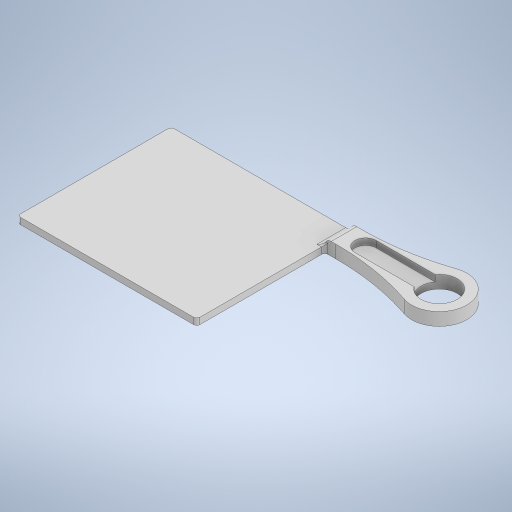
# Autodesk Inventor part: wachlarz
Saved by Autodesk Inventor 2023 (Build 270158000, 158)
## iProperties
Created: 2024-05-14
Part Number: wachlarz
Material: Ogólny
Document SubType Name: Modeling
Designer: kamil
Density: 1 g/cm^3
Appearance: Domyślna
Author: kamil
Autodesk Inventor part; units mm, degrees
ref_plane "YZ Plane" through (0, 0, 0) normal (1, 0, 0) x (0, 1, 0)
ref_plane "XZ Plane" through (0, 0, 0) normal (0, 1, 0) x (-1, 0, 0)
ref_plane "XY Plane" through (0, 0, 0) normal (0, 0, 1) x (1, 0, 0)
sketch "Szkic1" plane through (0, 0, 0) normal (0, 1, 0) x (-1, 0, 0)
  circle A0 centre (0, 0) radius 2.815
  circle A1 centre (0, 0) radius 4.315
  line L0 (43.875, 2) -> (0, 2)
  line L1 (0, 2) -> (0, -2)
  line L2 (0, -2) -> (43.875, -2)
  line L3 (43.875, -2) -> (43.875, 2)
  point P0 (43.875, 0)
  point P1 (3.8235, 2)
  point P2 (3.8235, -2)
  dimension "d0" = 5.63
  dimension "d2" = 1.5
  dimension "d5" = 43.875
  dimension "d6" = 4
  constraints: 8 end point, 2 centre point, 2 parallel, 1 coincident, 1 horizontal, 1 horizontal alignment, 1 midpoint, 1 perpendicular, 1 vertical alignment
  measures "d0" diameter of A0
  measures "d2" radial gap between concentric circles of A0 A1
  measures "d5" distance of L2.end L1.end
  measures "d6" distance of L1.end L0.end
extrude "Wyciągnięcie proste1" add sketch "Szkic1" along normal blind 2 contours A0 L0 A1 L2 | A0 L2 A1 L0 | L0 L3 L2 A1
sketch "Szkic2" plane through (0, 2, 0) normal (0, 1, 0) x (1, 0, 0)
  line L0 (-43.875, -2) -> (-3.8235, -2) projected
  arc A0 (-3.8235, -2) -> (-3.8235, 2) centre (0, 0) ccw projected
  line L1 (-3.8235, 2) -> (-43.875, 2) projected
  line L2 (-43.875, 2) -> (-43.875, -2) projected
  circle A1 centre (0, 0) radius 2.815 projected
  line L3 (-43.875, -2) -> (-15.875, -2)
  line L4 (-15.875, -2) -> (-15.875, -22)
  line L5 (-15.875, -22) -> (-43.875, -22)
  line L6 (-43.875, -22) -> (-43.875, -2)
  point P0 (-15.875, -2)
  dimension "d9" = 28
  dimension "d10" = 20
  constraints: 8 end point, 2 parallel, 1 horizontal, 1 perpendicular
  measures "d9" distance of L4.end L5.end
  measures "d10" distance of L3.end L4.end
extrude "Wyciągnięcie proste2" add sketch "Szkic2" against normal blind 2 contours L0 L4 L5 L6
sketch "Szkic3" plane through (0, 2, 0) normal (0, 1, 0) x (1, 0, 0)
  line L0 (0, 0) -> (-11.5, 0) construction
  line L1 (0, 1.65) -> (-11.5, 1.65)
  line L2 (-11.5, -1.65) -> (0, -1.65)
  arc A0 (0, -1.65) -> (0, 1.65) centre (0, 0) ccw
  arc A1 (-11.5, 1.65) -> (-11.5, -1.65) centre (-11.5, 0) ccw
  point P0 (-5.75, 0)
  dimension "d13" = 11.5
  dimension "d14" = 3.3
  constraints: 8 end point, 4 point on circle, 4 tangent, 2 centre point, 1 horizontal, 1 midpoint, 1 parallel
  measures "d13" distance of L0.start L0.end
  measures "d14" diameter of A1
extrude "Wyciągnięcie proste3" cut sketch "Szkic3" against normal blind 1
fillet "Zaokrąglenie1" radius 40 2 edges at (-3.8235, 1, 2) (-3.8235, 1, -2)
sketch "Szkic4" plane through (0, 2, 0) normal (0, 1, 0) x (1, 0, 0)
  line L0 (-2.2807, -1.65) -> (-11.5, -1.65) projected
  arc A0 (-11.5, 1.65) -> (-11.5, -1.65) centre (-11.5, 0) ccw projected
  line L1 (-11.5, 1.65) -> (-2.2807, 1.65) projected
  arc A1 (-2.2807, -1.65) -> (-2.2807, 1.65) centre (0, 0) ccw projected
  line L2 (-15.875, -2) -> (-14.1357, -2) projected
  arc A2 (-1.3764, -4.0896) -> (-14.1357, -2) centre (-14.1357, -42) ccw projected
  arc A3 (-1.3764, -4.0896) -> (-1.3764, 4.0896) centre (0, 0) ccw projected
  arc A4 (-14.1357, 2) -> (-1.3764, 4.0896) centre (-14.1357, 42) ccw projected
  line L3 (-14.1357, 2) -> (-43.875, 2) projected
  line L4 (-43.875, 2) -> (-43.875, -22) projected
  line L5 (-43.875, -22) -> (-15.875, -22) projected
  line L6 (-15.875, -22) -> (-15.875, -2) projected
  line L7 (-15.875, -2) -> (-15.875, 2)
  constraints: 2 end point, 1 perpendicular, 1 point on line
extrude "Wyciągnięcie proste4" cut sketch "Szkic4" against normal blind 1 contours L6 L5 L4 L3 L7
fillet "Zaokrąglenie2" radius 1 2 edges at (-15.875, 2, 0) (-15.875, 1, 0)
fillet "Zaokrąglenie3" radius 0.5 5 edges at (-15.875, 0.5, 22) (-43.875, 0.5, 22) (-43.875, 0.5, -2) (-15.875, 0.5, 2) (-16.241, 1, 2)
